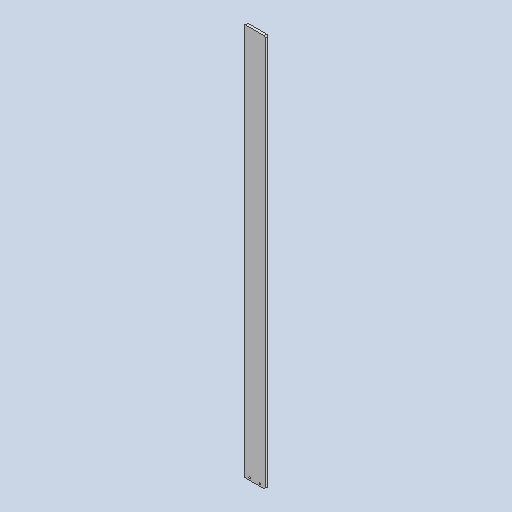
# Autodesk Inventor part: Фанерка хвоста
Saved by Autodesk Inventor 2023.2 (Build 272271030, 271C)
## iProperties
Created: 2024-03-12
Part Number: Фанерка хвоста
Material: Типовые
Document SubType Name: Modeling
Designer: I9232
Density: 1 g/cm^3
Appearance: По умолчанию
Author: I9232
Autodesk Inventor part; units mm, degrees
ref_plane "YZ Plane" through (0, 0, 0) normal (1, 0, 0) x (0, 1, 0)
ref_plane "XZ Plane" through (0, 0, 0) normal (0, 1, 0) x (-1, 0, 0)
sketch "Эскиз1" plane through (0, 0, 0) normal (0, 0, 1) x (1, 0, 0)
  line L0 (-16, -300) -> (16, -300)
  line L1 (16, -300) -> (16, 300)
  line L2 (16, 300) -> (-16, 300)
  line L3 (-16, 300) -> (-16, -300)
  line L4 (-16, -300) -> (16, 300) construction
  line L5 (16, -300) -> (-16, 300) construction
  point P0 (0, 0)
  dimension "d0" = 600
  dimension "d1" = 32
  constraints: 12 end point, 2 midpoint, 2 parallel, 1 horizontal, 1 perpendicular
  measures "d0" distance of L0.end L1.end
  measures "d1" distance of L1.end L2.end
extrude "Выдавливание1" add sketch "Эскиз1" along normal mid plane 4
fillet "Сопряжение1" radius 2 4 edges at (-16, -300, 0) (16, -300, 0) (16, 300, 0) (-16, 300, 0)
sketch "Эскиз3" plane through (0, 0, 2) normal (0, 0, 1) x (1, 0, 0)
  circle A0 centre (-8, -296.75) radius 1.25 projected
  circle A1 centre (8, -296.75) radius 1.25 projected
  point P0 (0, 0)
ref_plane "РабПлоскость1" through (-309.8315, -315.671, -2) normal (0, 0, 1) x (1, 0, 0)
extrude "Выдавливание3" cut sketch "Эскиз3" against normal up to surface (4 mm away)
